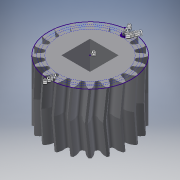
# Autodesk Inventor part: gear 4 shaft herring
Saved by Autodesk Inventor 2017 (Build 210142000, 142)
## iProperties
Created: 2018-04-17
Part Number: gear 4 shaft herring
Material: Generic
Document SubType Name: Modeling
Designer: RKL
Density: 1 g/cm^3
Appearance: Default
Author: RKL
Autodesk Inventor part; units mm, degrees
ref_plane "YZ Plane" through (0, 0, 0) normal (1, 0, 0) x (0, 1, 0)
ref_plane "XZ Plane" through (0, 0, 0) normal (0, 1, 0) x (-1, 0, 0)
ref_plane "XY Plane" through (0, 0, 0) normal (0, 0, 1) x (1, 0, 0)
sketch "Sketch1" plane through (0, 0, 0) normal (0, 0, 1) x (1, 0, 0)
  spline S0 degree 3 poles (-1.834935, 13.624531) (-1.724023, 13.481558) (-1.502208, 13.195624) (-1.21737, 12.732418) (-1.021921, 12.324056) (-0.897506, 11.983424) (-0.8637, 11.80555) (-0.846805, 11.716656) knots 0 0 0 0 0.25005583 0.50009345 0.75006675 0.87509433 1 1 1 1
  spline S1 degree 3 poles (-0.846805, 11.716656) (-0.834304, 11.588536) (-0.815551, 11.396339) (-0.740419, 11.149746) (-0.655636, 10.975759) (-0.53515, 10.823162) (-0.378871, 10.707427) (-0.193463, 10.641766) (0, 10.646798) (0.193463, 10.641766) (0.378871, 10.707427) (0.53515, 10.823162) (0.655636, 10.975759) (0.740419, 11.149746) (0.815551, 11.396339) (0.834304, 11.588536) (0.846805, 11.716656) knots 0 0 0 0 0.12504484 0.18758265 0.25015403 0.31267057 0.37510908 0.43748213 0.5 0.56251787 0.62489092 0.68732943 0.74984597 0.81241735 0.87495516 1 1 1 1
  spline S2 degree 3 poles (0.846805, 11.716656) (0.8637, 11.80555) (0.897506, 11.983424) (1.021921, 12.324056) (1.21737, 12.732418) (1.502208, 13.195624) (1.724023, 13.481558) (1.834935, 13.624531) knots 0 0 0 0 0.12490567 0.24993325 0.49990655 0.74994417 1 1 1 1
  circle A0 centre (0, 0) radius 10.64512 construction
  circle A1 centre (0, 0) radius 11.746158 construction
  circle A2 centre (0, 0) radius 12.5 construction
  circle A3 centre (0, 0) radius 13.747539
  point P0 (-1.510176, 13.189888)
  point P1 (-1.225729, 12.727904)
  point P2 (-0.993485, 12.237749)
  point P3 (-0.904582, 11.981446)
  point P4 (-0.7926, 11.335532)
  point P5 (-0.735692, 11.151607)
  point P6 (-0.649644, 10.979263)
  point P7 (-0.529102, 10.829226)
  point P8 (-0.373959, 10.715736)
  point P9 (-0.19228, 10.653572)
  point P10 (0, 10.64512)
  point P11 (0.19228, 10.653572)
  point P12 (0.373959, 10.715736)
  point P13 (0.529102, 10.829226)
  point P14 (0.649644, 10.979263)
  point P15 (0.735692, 11.151607)
  point P16 (0.7926, 11.335532)
  point P17 (0.904582, 11.981446)
  point P18 (0.993485, 12.237749)
  point P19 (1.225729, 12.727904)
  point P20 (1.510176, 13.189888)
  constraints: 4 centre point, 2 point on circle, 57 other
extrude "Extrusion1" add sketch "Sketch1" against normal blind 20
extrude "Extrusion2" [suppressed]
pattern_circular "Circular Pattern1" [suppressed]
sketch "Sketch2" plane through (0, 0, 0) normal (0, 0, 1) x (1, 0, 0)
  line L0 (4.7625, -4.7625) -> (-4.7625, -4.7625)
  line L1 (-4.7625, -4.7625) -> (-4.7625, 4.7625)
  line L2 (-4.7625, 4.7625) -> (4.7625, 4.7625)
  line L3 (4.7625, 4.7625) -> (4.7625, -4.7625)
  line L4 (4.7625, -4.7625) -> (-4.7625, 4.7625) construction
  line L5 (-4.7625, -4.7625) -> (4.7625, 4.7625) construction
  point P0 (0, 0)
  dimension "d7" = 9.525
  constraints: 12 end point, 2 midpoint, 2 parallel, 2 perpendicular, 1 horizontal
  measures "d7" distance of L0.end L1.end
extrude "Extrusion3" cut sketch "Sketch2" against normal through all
coil "Coil1" sketch "Sketch1" operation cut axis through (0, 0, -10) along (0, 0, -1) pitch 1000 turns 0.01 hand right contours A3 S2 S1 S0
sketch "Sketch3" plane through (0, 0, -10) normal (0, 0, 1) x (0.9980267, -0.0627905, 0)
  spline S0 degree 3 poles (-0.846805, 11.716656) (-0.8637, 11.80555) (-0.897506, 11.983424) (-1.021921, 12.324056) (-1.21737, 12.732418) (-1.502208, 13.195624) (-1.724023, 13.481558) (-1.834935, 13.624531) knots 0 0 0 0 0.12490567 0.24993325 0.49990655 0.74994417 1 1 1 1
  spline S1 degree 3 poles (0.846805, 11.716656) (0.834304, 11.588536) (0.815551, 11.396339) (0.740419, 11.149746) (0.655636, 10.975759) (0.53515, 10.823162) (0.378871, 10.707427) (0.193463, 10.641766) (0, 10.646798) (-0.193463, 10.641766) (-0.378871, 10.707427) (-0.53515, 10.823162) (-0.655636, 10.975759) (-0.740419, 11.149746) (-0.815551, 11.396339) (-0.834304, 11.588536) (-0.846805, 11.716656) knots 0 0 0 0 0.12504484 0.18758265 0.25015403 0.31267057 0.37510908 0.43748213 0.5 0.56251787 0.62489092 0.68732943 0.74984597 0.81241735 0.87495516 1 1 1 1
  spline S2 degree 3 poles (1.834935, 13.624531) (1.724023, 13.481558) (1.502208, 13.195624) (1.21737, 12.732418) (1.021921, 12.324056) (0.897506, 11.983424) (0.8637, 11.80555) (0.846805, 11.716656) knots 0 0 0 0 0.25005583 0.50009345 0.75006675 0.87509433 1 1 1 1
  arc A0 (1.834935, 13.624531) -> (-1.834935, 13.624531) centre (0, 0) ccw
  constraints: 1 horizontal alignment, 2 other
coil "Coil2" sketch "Sketch3" operation cut axis through (0, 0, -10) along (0, 0, -1) pitch 1000 turns 0.01 hand left
pattern_circular "Circular Pattern2" count 20 over 360 about axis through (0, 0, 0) along (0, 0, -1) of "Coil1", "Coil2"
equation "\"d0\" = FaceWidth"
equation "\"Module\" = 1.25"
equation "\"PressureAngle\" = 20deg"
equation "\"UnitProfileClearance\" = 0.25"
equation "\"UnitRoundRadius\" = 0.35"
equation "\"HeadDiameter\" = 27.49508"
equation "\"RootDiameter\" = 21.29024"
equation "\"BaseDiameter\" = 23.49232"
equation "\"PitchDiameter\" = 25"
equation "\"FaceWidth\" = 20"
equation "\"HelixAngle\" = 0"
equation "\"UnitCorrection\" = 0"
equation "\"UnitAddendumModification\" = 0.001969"
equation "\"CircularPitch\" = 3.926991"
equation "\"UnitBacklashShift\" = -0.233904"
equation "\"TotalToolShift\" = -0.29238"
equation "\"IsInternal\" = 0"
body "Solid1"
